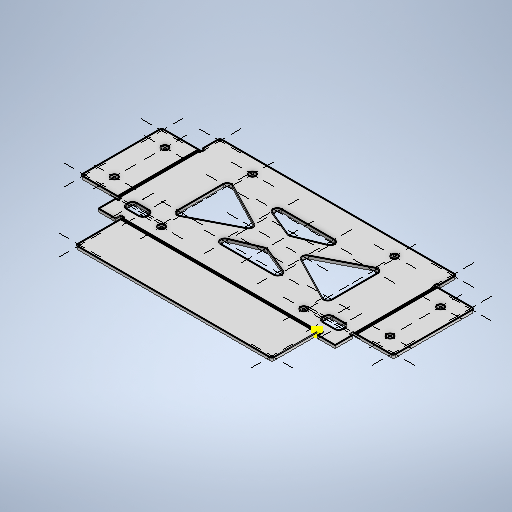
# Autodesk Inventor part: body_back_frame
Saved by Autodesk Inventor 2026.1 (Build 301233000, 233)
## iProperties
Created: 2025-08-16
Part Number: body_back_frame
Material: Generic
Document SubType Name: Modeling
Designer: chris
Density: 1 g/cm^3
Appearance: Default
Author: chris
Autodesk Inventor part; units mm, degrees
ref_plane "YZ Plane" through (0, 0, 0) normal (1, 0, 0) x (0, 1, 0)
ref_plane "XZ Plane" through (0, 0, 0) normal (0, 1, 0) x (-1, 0, 0)
ref_plane "XY Plane" through (0, 0, 0) normal (0, 0, 1) x (1, 0, 0)
sketch "Sketch1" plane through (0, 0, 0) normal (0, 1, 0) x (-1, 0, 0)
  line L0 (97, -0.4496) -> (0, -0.4496)
  line L1 (-10.1396, -9.0893) -> (-10.1396, -49.0893)
  line L2 (107.1396, -49.0893) -> (107.1396, -9.0893)
  circle A0 centre (83.69, -51.8993) radius 1.55
  circle A1 centre (13.31, -51.8993) radius 1.55
  circle A2 centre (83.69, -6.8993) radius 1.55
  circle A3 centre (13.31, -6.8993) radius 1.55
  arc A4 (5, -7.8993) -> (3, -5.8993) centre (3, -7.8993) ccw
  line L3 (-3, -5.8993) -> (3, -5.8993)
  arc A5 (3, -10.8993) -> (5, -8.8993) centre (3, -8.8993) ccw
  line L4 (5, -7.8993) -> (5, -8.8993)
  arc A6 (-5, -8.8993) -> (-3, -10.8993) centre (-3, -8.8993) ccw
  line L5 (-5, -8.8993) -> (-5, -7.8993)
  arc A7 (-3, -5.8993) -> (-5, -7.8993) centre (-3, -7.8993) ccw
  arc A8 (100, -10.8993) -> (102, -8.8993) centre (100, -8.8993) ccw
  line L6 (102, -7.8993) -> (102, -8.8993)
  arc A9 (92, -8.8993) -> (94, -10.8993) centre (94, -8.8993) ccw
  line L7 (92, -8.8993) -> (92, -7.8993)
  arc A10 (102, -7.8993) -> (100, -5.8993) centre (100, -7.8993) ccw
  line L8 (94, -5.8993) -> (100, -5.8993)
  arc A11 (94, -5.8993) -> (92, -7.8993) centre (94, -7.8993) ccw
  arc A12 (13.2291, -16.0132) -> (10.31, -17.7895) centre (12.31, -17.7895) ccw
  line L9 (10.31, -40.389) -> (10.31, -17.7895)
  arc A13 (35.0671, -30.8656) -> (35.0671, -27.313) centre (34.148, -29.0893) ccw
  line L10 (13.2291, -16.0132) -> (35.0671, -27.313)
  arc A14 (10.31, -40.389) -> (13.2291, -42.1653) centre (12.31, -40.389) ccw
  line L11 (35.0671, -30.8656) -> (13.2291, -42.1653)
  arc A15 (34.6713, -40.2421) -> (35.4379, -44.0893) centre (35.4379, -42.0893) ccw
  line L12 (34.6713, -40.2421) -> (47.7334, -34.821)
  arc A16 (61.5621, -44.0893) -> (62.3287, -40.2421) centre (61.5621, -42.0893) ccw
  line L13 (49.2666, -34.821) -> (62.3287, -40.2421)
  arc A17 (49.2666, -34.821) -> (47.7334, -34.821) centre (48.5, -36.6682) ccw
  arc A18 (61.9329, -27.313) -> (61.9329, -30.8656) centre (62.852, -29.0893) ccw
  line L14 (61.9329, -27.313) -> (83.7709, -16.0132)
  arc A19 (86.69, -17.7895) -> (83.7709, -16.0132) centre (84.69, -17.7895) ccw
  line L15 (86.69, -17.7895) -> (86.69, -40.389)
  arc A20 (83.7709, -42.1653) -> (86.69, -40.389) centre (84.69, -40.389) ccw
  arc A21 (47.7334, -23.3576) -> (49.2666, -23.3576) centre (48.5, -21.5104) ccw
  line L16 (62.3287, -17.9365) -> (49.2666, -23.3576)
  arc A22 (62.3287, -17.9365) -> (61.5621, -14.0893) centre (61.5621, -16.0893) ccw
  line L17 (35.4379, -14.0893) -> (61.5621, -14.0893)
  arc A23 (35.4379, -14.0893) -> (34.6713, -17.9365) centre (35.4379, -16.0893) ccw
  line L18 (47.7334, -23.3576) -> (34.6713, -17.9365)
  line L19 (100, -10.8993) -> (94, -10.8993)
  line L20 (3, -10.8993) -> (-3, -10.8993)
  circle A24 centre (-19.6843, -41.5893) radius 1.55
  circle A25 centre (116.6843, -41.5893) radius 1.55
  circle A26 centre (-19.6843, -16.5893) radius 1.55
  circle A27 centre (116.6843, -16.5893) radius 1.55
  line L21 (83.7709, -42.1653) -> (61.9329, -30.8656)
  line L22 (61.5621, -44.0893) -> (35.4379, -44.0893)
  arc A28 (124.7793, -49.0893) -> (125.7793, -48.0893) centre (124.7793, -48.0893) ccw
  line L23 (125.7793, -10.0893) -> (125.7793, -48.0893)
  arc A29 (125.7793, -10.0893) -> (124.7793, -9.0893) centre (124.7793, -10.0893) ccw
  arc A30 (97, 21.19) -> (96, 22.19) centre (96, 21.19) ccw
  line L24 (1, 22.19) -> (96, 22.19)
  arc A31 (106, -59.0893) -> (107, -58.0893) centre (106, -58.0893) ccw
  line L25 (106, -59.0893) -> (-9, -59.0893)
  arc A32 (-10, -58.0893) -> (-9, -59.0893) centre (-9, -58.0893) ccw
  arc A33 (-28.7793, -48.0893) -> (-27.7793, -49.0893) centre (-27.7793, -48.0893) ccw
  arc A34 (-27.7793, -9.0893) -> (-28.7793, -10.0893) centre (-27.7793, -10.0893) ccw
  line L26 (-27.7793, -9.0893) -> (-8.94, -9.0893)
  arc A35 (1, 22.19) -> (0, 21.19) centre (1, 21.19) ccw
  line L27 (124.7793, -49.0893) -> (105.94, -49.0893)
  line L28 (-28.7793, -48.0893) -> (-28.7793, -10.0893)
  line L29 (107, -50.5893) -> (105.94, -50.5893)
  line L30 (105.94, -50.5893) -> (105.94, -49.0893)
  line L31 (107, -50.5893) -> (107, -58.0893)
  line L32 (105.94, -7.5893) -> (107, -7.5893)
  line L33 (105.94, -9.0893) -> (124.7793, -9.0893)
  line L34 (105.94, -9.0893) -> (105.94, -7.5893)
  line L35 (107, 0.9107) -> (107, -7.5893)
  line L36 (-10, -7.5893) -> (-8.94, -7.5893)
  line L37 (-8.94, -7.5893) -> (-8.94, -9.0893)
  line L38 (-10, -7.5893) -> (-10, 0.9107)
  line L39 (-8.94, -50.5893) -> (-10, -50.5893)
  line L40 (-8.94, -49.0893) -> (-27.7793, -49.0893)
  line L41 (-8.94, -49.0893) -> (-8.94, -50.5893)
  line L42 (-10, -58.0893) -> (-10, -50.5893)
  line L43 (97, 21.19) -> (97, -1.6493)
  line L44 (0, 21.19) -> (0, -1.6493)
  line L45 (0, -1.6493) -> (-1.5, -1.6493)
  line L46 (-1.5, -1.6493) -> (-1.5, 0.9107)
  line L47 (-10, 0.9107) -> (-1.5, 0.9107)
  line L48 (98.5, 0.9107) -> (107, 0.9107)
  line L49 (98.5, 0.9107) -> (98.5, -1.6493)
  line L50 (98.5, -1.6493) -> (97, -1.6493)
  line L51 (107.5893, -9.0893) -> (107.5893, -49.0893)
  line L52 (-10.5893, -49.0893) -> (-10.5893, -9.0893)
  line L53 (106.69, -49.0893) -> (106.69, -9.0893)
  line L54 (-9.69, -9.0893) -> (-9.69, -49.0893)
  line L55 (97, -0.8993) -> (0, -0.8993)
  line L56 (0, 0) -> (97, 0)
  constraints: 114 end point, 65 tangent, 56 point on circle, 36 centre point, 33 equal radius, 27 parallel, 26 vertical, 23 horizontal, 22 perpendicular, 18 point on line, 175 other
extrude "Extrusion1" add sketch "Sketch1" against normal blind 1.5
body "Solid1"
